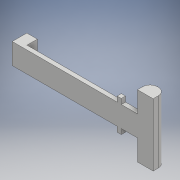
# Autodesk Inventor part: gravity_holder
Saved by Autodesk Inventor 2017 (Build 210142000, 142)
## iProperties
Created: 2016-06-06
Part Number: gravity_holder
Material: Generic
Document SubType Name: Modeling
Designer: Conor
Density: 1 g/cm^3
Appearance: Default
Author: Conor
Autodesk Inventor part; units mm, degrees
ref_plane "YZ Plane" through (0, 0, 0) normal (1, 0, 0) x (0, 1, 0)
ref_plane "XZ Plane" through (0, 0, 0) normal (0, 1, 0) x (-1, 0, 0)
ref_plane "XY Plane" through (0, 0, 0) normal (0, 0, 1) x (1, 0, 0)
sketch "rod" plane through (0, 0, 0) normal (0, 1, 0) x (-1, 0, 0)
  line L0 (8.8103, 11.8971) -> (-111.1897, 11.8971)
  line L1 (-111.1897, 11.8971) -> (-111.1897, -8.1029)
  line L2 (-111.1897, -8.1029) -> (8.8103, -8.1029)
  line L3 (8.8103, -8.1029) -> (8.8103, 11.8971)
  point P0 (0, 0)
  dimension "d0" = 20
  dimension "d1" = 120
  constraints: 8 end point, 2 parallel, 1 horizontal, 1 perpendicular
  measures "d0" distance of L2.end L0.start
  measures "d1" distance of L1.end L2.end
extrude "Extrusion1" add sketch "rod" along normal blind 4
sketch "Sketch2" plane through (0, 0, 0) normal (0, -1, 0) x (1, 0, 0)
  line L0 (111.1897, 31.8971) -> (126.1897, 31.8971)
  line L1 (126.1897, 31.8971) -> (126.1897, -28.1029)
  line L2 (126.1897, -28.1029) -> (111.1897, -28.1029)
  line L3 (111.1897, -28.1029) -> (111.1897, 31.8971)
  line L4 (111.1897, 11.8971) -> (111.1897, -8.1029) projected
  line L5 (-8.8103, 11.8971) -> (111.1897, 11.8971) projected
  point P0 (0, 0)
  dimension "d6" = 15
  dimension "d7" = 60
  dimension "d8" = 20
  constraints: 8 end point, 2 parallel, 1 collinear, 1 horizontal, 1 perpendicular
  measures "d6" distance of L0.start L0.end
  measures "d7" distance of L0.end L1.end
  measures "d8" distance between parallel lines of L0 L5
extrude "Extrusion2" add sketch "Sketch2" against normal blind 12
fillet "Fillet1" radius 7 2 edges at (111.1897, 12, 1.8971) (126.1897, 12, 1.8971)
sketch "Sketch3" plane through (0, 4, 0) normal (0, 1, 0) x (1, 0, 0)
  line L0 (-8.8103, -11.8971) -> (111.1897, -11.8971) projected
  line L1 (111.1897, 8.1029) -> (-8.8103, 8.1029) projected
  line L2 (-8.8103, -11.8971) -> (1.2928, -11.8971)
  line L3 (1.2928, -11.8971) -> (1.2928, 8.1029)
  line L4 (1.2928, 8.1029) -> (-8.8103, 8.1029)
  line L5 (-8.8103, 8.1029) -> (-8.8103, -11.8971)
  point P0 (0, 0)
  constraints: 8 end point, 2 parallel, 1 horizontal, 1 perpendicular, 1 point on line
extrude "Extrusion3" add sketch "Sketch3" along normal blind 10
sketch "Sketch4" plane through (0, 14, 0) normal (0, 1, 0) x (1, 0, 0)
  circle A0 centre (-7.6103, -1.8971) radius 0.5166
  circle A1 centre (-5.0911, -1.8971) radius 1.0075
  circle A2 centre (-1.4334, -1.8971) radius 1.5342
  line L0 (-8.8103, -11.8971) -> (1.2928, -11.8971) projected
  line L1 (-8.8103, 8.1029) -> (-8.8103, -11.8971) projected
  point P0 (0, 0)
  dimension "d14" = 10
  dimension "d15" = 10
  dimension "d16" = 10
  dimension "d17" = 10.1031
  dimension "d18" = 1.2
  constraints: 3 centre point
  measures "d14" distance from line of L0 A2.centre
  measures "d15" distance from line of L0 A1.centre
  measures "d16" distance from line of L0 A0.centre
  measures "d17" distance of L0.start L0.end
  measures "d18" distance from line of L1 A0.centre
extrude "Extrusion4" cut sketch "Sketch4" against normal blind 11.5
sketch "Sketch5" plane through (111.1897, 0, -8.1029) normal (0, 0, -1) x (-1, 0, 0)
  line L0 (0, 4) -> (109.8969, 4) projected
  line L1 (120, 0) -> (0, 0) projected
  line L2 (19.4969, 4) -> (15.4969, 4)
  line L3 (15.4969, 4) -> (15.4969, 0)
  line L4 (15.4969, 0) -> (19.4969, 0)
  line L5 (19.4969, 0) -> (19.4969, 4)
  line L6 (109.8969, 4) -> (109.8969, 14) projected
  point P0 (111.1897, 0)
  dimension "d23" = 4
  dimension "d24" = 90.4
  constraints: 8 end point, 2 parallel, 2 point on line, 1 horizontal, 1 perpendicular
  measures "d23" distance between parallel lines of L5 L3
  measures "d24" distance between parallel lines of L6 L5
extrude "Extrusion5" add sketch "Sketch5" along normal blind 5
sketch "Sketch6" plane through (-8.8103, 0, 11.8971) normal (0, 0, 1) x (1, 0, 0)
  line L0 (100.5031, 4) -> (10.1031, 4) projected
  line L1 (100.5031, 0) -> (0, 0) projected
  line L2 (104.5031, 4) -> (100.5031, 4)
  line L3 (100.5031, 4) -> (100.5031, 0)
  line L4 (100.5031, 0) -> (104.5031, 0)
  line L5 (104.5031, 0) -> (104.5031, 4)
  line L6 (10.1031, 4) -> (10.1031, 14) projected
  point P0 (8.8103, 0)
  dimension "d27" = 4
  dimension "d28" = 90.4
  constraints: 8 end point, 2 parallel, 2 point on line, 1 horizontal, 1 perpendicular
  measures "d27" distance between parallel lines of L5 L3
  measures "d28" distance between parallel lines of L3 L6
extrude "Extrusion6" add sketch "Sketch6" along normal blind 5
equation "\"d8\" = 0.25 * d7 + 0.25 * d0"
equation "\"d14\" = 0.5 * d0"
equation "\"d15\" = d14"
equation "\"d16\" = d14"
body "Solid1"
